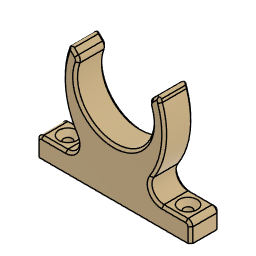
Prendedor de escada v6 (Autodesk Fusion 360 design; units mm, degrees)
Autodesk Fusion 360 part; units mm, degrees
sketch "Sketch1" plane through (0, 0, 0) normal (0, 1, 0) x (1, 0, 0)
  circle A0 centre (0, 0) radius 16
  arc A1 (-15.7781, 20.2968) -> (-19.3265, -8.4635) centre (12.3363, 2.229) ccw
  arc A2 (-15.576, -8.2055) -> (-15, -5.5678) centre (-17.3437, -6.4377) ccw
  arc A3 (-15.7781, 20.2968) -> (-19.9844, 28) centre (-19.9844, 23) ccw
  line L0 (-19.9844, 28) -> (-31.9844, 28)
  line L1 (-31.9844, 28) -> (-31.9844, 36)
  line L2 (-31.9844, 36) -> (31.9844, 36)
  line L3 (0, 0) -> (0, -16) construction
  line L4 (0, 16) -> (0, 36) construction
  line L5 (0, 16) -> (0, 0) construction
  line L6 (31.9844, 28) -> (31.9844, 36)
  line L7 (19.9844, 28) -> (31.9844, 28)
  arc A4 (19.9844, 28) -> (15.7781, 20.2968) centre (19.9844, 23) ccw
  arc A5 (19.3265, -8.4635) -> (15.7781, 20.2968) centre (-12.3363, 2.229) ccw
  line L8 (-15.576, -8.2055) -> (-17.6973, -10.3268)
  line L9 (-19.3265, -8.4635) -> (-18.6973, -10.3268)
  line L10 (-17.6973, -10.3268) -> (-18.6973, -10.3268)
  arc A6 (15, -5.5678) -> (15.576, -8.2055) centre (17.3437, -6.4377) ccw
  line L11 (15.576, -8.2055) -> (17.6973, -10.3268)
  line L12 (17.6973, -10.3268) -> (18.6973, -10.3268)
  line L13 (19.3265, -8.4635) -> (18.6973, -10.3268)
  line L14 (16, 0) -> (16, -7.5757) construction
  dimension "d1" = 32
  dimension "d3" = 2.5
  dimension "d4" = 8
  dimension "d5" = 12
  dimension "d6" = 5
  dimension "d10" = 20
  dimension "d22" = 1
  dimension "d23" = 3
  dimension "d24" = 30
  dimension "d25" = 45
  dimension "d28" = 1
  constraint coincident A0.centre L3.start
  constraint tangent A0 A2
  constraint coincident A0 A2.end
  constraint tangent A1 A2
  constraint tangent A1 A3
  constraint horizontal L0
  constraint perpendicular L0 L1
  constraint perpendicular L1 L2
  constraint coincident A0 L3.end
  constraint vertical L3
  constraint tangent A3 L0
  constraint coincident A0 L4.start
  constraint coincident L2 L4.end
  constraint midpoint L2 L4.end
  constraint vertical L4
  constraint vertical L5
  constraint symmetric A1.end L5 A5.start
  constraint symmetric A1.start L5 A4.end
  constraint symmetric A1 L5 A5
  constraint symmetric A3.end L5 L7.start
  constraint symmetric A3 L5 A4
  constraint symmetric L0.end L5 L6.start
  constraint symmetric L1.end L5 L2.end
  constraint tangent A2 L8
  constraint tangent A1 L9
  constraint horizontal L10
  constraint symmetric A1.end L3 A5.start
  constraint symmetric A2.end L3 A6.start
  constraint symmetric A2 L3 A6
  constraint symmetric L3 A2.start A6.end
  constraint symmetric L3 L8.end L11.end
  constraint symmetric L3 L9.end L12.end
  constraint coincident A0 L14.start
  constraint vertical L14
  constraint tangent A0 L14
  measures "d1" diameter of A0
  measures "d3" radius of A2
  measures "d4" distance of L0.end L1.end
  measures "d5" distance of A3.end L0.end
  measures "d6" radius of A3
  measures "d10" distance of L4.start L4.end
  measures "d22" distance of L8.end L9.end
  measures "d23" distance of A2.start L8.end
  measures "d24" distance of A2.end A6.start
  measures "d25" angle of L3 L8
  measures "d28" distance of A6.start L14
extrude "Extrude1" add sketch "Sketch1" along normal blind 12 contours A0 A1 A2 A3 L0 L1 L2 L6 L7 A4 A5 L8 L9 L10 A6 L11 L12 L13
fillet "Fillet1" radius 2 2 edges at (-31.9844, 6, -28) (31.9844, 6, -28)
chamfer "Chamfer1" distance 1 angle 45 34 edges at (-20.8317, 0, -6.3213) (-15.596, 0, -25.3963) (-24.9844, 0, -28) (-31.3986, 0, -28.5858) (-31.9844, 0, -33) (-19.0119, 0, 9.3952) (-14.9013, 0, 6.9711) (-16.6366, 0, 9.2662) (16.6366, 0, 9.2662) (14.9013, 0, 6.9711) (0, 0, -16) (20.8317, 0, -6.3213) (19.0119, 0, 9.3952) (31.9844, 0, -33) (31.3986, 0, -28.5858) (24.9844, 0, -28) (15.596, 0, -25.3963) (-20.8317, 12, -6.3213) (-15.596, 12, -25.3963) (-24.9844, 12, -28) (-31.3986, 12, -28.5858) (-31.9844, 12, -33) (-19.0119, 12, 9.3952) (-14.9013, 12, 6.9711) (-16.6366, 12, 9.2662) (16.6366, 12, 9.2662) (14.9013, 12, 6.9711) (0, 12, -16) (20.8317, 12, -6.3213) (19.0119, 12, 9.3952) (31.9844, 12, -33) (31.3986, 12, -28.5858) (24.9844, 12, -28) (15.596, 12, -25.3963)
sketch "Sketch2" plane through (0, 0, -28) normal (0, 0, 1) x (-1, 0, 0)
  line L0 (19.9844, -11) -> (29.9844, -11)
  line L1 (29.9844, -11) -> (29.9844, -1)
  line L2 (29.9844, -1) -> (19.9844, -1)
  line L3 (19.9844, -1) -> (19.9844, -11)
  line L4 (-29.9844, -11) -> (-19.9844, -11)
  line L5 (-19.9844, -11) -> (-19.9844, -1)
  line L6 (-19.9844, -1) -> (-29.9844, -1)
  line L7 (-29.9844, -1) -> (-29.9844, -11)
  line L8 (29.9844, -11) -> (19.9844, -1) construction
  circle A0 centre (24.9844, -6) radius 1.75
  line L9 (-29.9844, -1) -> (-19.9844, -11) construction
  circle A1 centre (-24.9844, -6) radius 1.75
  dimension "d16" = 3.5
  constraint coincident L0.end L1.start
  constraint coincident L2.end L3.start
  constraint midpoint L8 A0.centre
  constraint coincident L6.end L7.start
  constraint coincident L4.end L5.start
  constraint midpoint L9 A1.centre
  constraint equal A0 A1
  measures "d16" diameter of A0
extrude "Extrude2" cut sketch "Sketch2" against normal blind 14 contours A0 | A1
chamfer "Chamfer2" distance 2 angle 45 2 edges at (26.616, 5.3672, -28) (-23.3528, 5.3672, -28)
fillet "Fillet2" radius 1 4 edges at (-18.6973, 6, 10.3268) (-17.6973, 6, 10.3268) (17.6973, 6, 10.3268) (18.6973, 6, 10.3268)
extrude "Extrude3" [suppressed]
